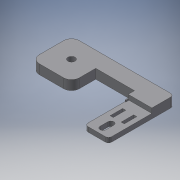
# Autodesk Inventor part: FiberMount
Saved by Autodesk Inventor 2019 (Build 230136000, 136)
## iProperties
Created: 2019-05-24
Part Number: FiberMount
Material: Generic
Document SubType Name: Modeling
Designer: aorfi
Density: 1 g/cm^3
Appearance: Default
Author: aorfi
Autodesk Inventor part; units mm, degrees
ref_plane "YZ Plane" through (0, 0, 0) normal (1, 0, 0) x (0, 1, 0)
ref_plane "XZ Plane" through (0, 0, 0) normal (0, 1, 0) x (-1, 0, 0)
ref_plane "XY Plane" through (0, 0, 0) normal (0, 0, 1) x (1, 0, 0)
sketch "Sketch1" plane through (0, 0, 0) normal (0, 1, 0) x (-1, 0, 0)
  line L0 (-7.5, 25) -> (7.5, 25)
  line L1 (7.5, 25) -> (7.5, -16.5)
  line L2 (7.5, -16.5) -> (-7.5, -16.5)
  line L3 (-7.5, -16.5) -> (-7.5, 25)
  line L4 (7.5, -16.5) -> (57.5, -16.5)
  line L5 (57.5, -16.5) -> (57.5, 8.9)
  line L6 (57.5, 8.9) -> (32.1, 8.9)
  line L7 (32.1, 8.9) -> (32.1, -6.5)
  line L8 (32.1, -6.5) -> (7.5, -6.5)
  point P0 (0, 0)
  point P1 (0, -16.5)
  point P2 (57.5, -3.8)
  dimension "d30" = 15
  dimension "d31" = 16.5
  dimension "d32" = 25
  dimension "d59" = 50
  dimension "d60" = 25.4
  dimension "d61" = 10
  dimension "d62" = 25.4
  constraints: 18 end point, 4 horizontal, 3 perpendicular, 2 midpoint, 2 parallel, 1 point on line, 1 vertical alignment
  measures "d30" distance of L0.start L0.end
  measures "d31" distance from line of L2 point (0, 0)
  measures "d32" distance from line of point (0, 0) L0
  measures "d59" distance between parallel lines of L5 L1
  measures "d60" distance between parallel lines of L4 L6
  measures "d61" distance between parallel lines of L4 L8
  measures "d62" distance between parallel lines of L5 L7
extrude "Extrusion1" add sketch "Sketch1" along normal mid plane 3
sketch "Sketch4" plane through (0, 1.5, 0) normal (0, 1, 0) x (1, 0, 0)
  line L0 (7.5, 2.5) -> (-7.5, 2.5)
  line L1 (7.5, 2.5) -> (7.5, 14.5)
  line L2 (-7.5, 6.5) -> (-7.5, 2.5)
  line L3 (7.5, -25) -> (7.5, 16.5) projected
  line L4 (-7.5, 6.5) -> (-7.5, -25) projected
  line L5 (-7.5, -25) -> (7.5, -25) projected
  line L6 (7.5, 16.5) -> (-57.5, 16.5) projected
  line L7 (7.5, 16.5) -> (-7.5, 16.5)
  line L8 (-7.5, -25) -> (7.5, -25) projected
  line L9 (7.5, -25) -> (7.5, 16.5) projected
  line L10 (7.5, 16.5) -> (-57.5, 16.5) projected
  line L11 (-57.5, 16.5) -> (-57.5, -8.9) projected
  line L12 (-57.5, -8.9) -> (-32.1, -8.9) projected
  line L13 (-32.1, -8.9) -> (-32.1, 6.5) projected
  line L14 (-32.1, 6.5) -> (-7.5, 6.5) projected
  line L15 (-7.5, 6.5) -> (-7.5, -25) projected
  point P0 (0, 0)
  dimension "d20" = 2.5
  constraints: 8 end point, 2 collinear, 2 horizontal, 2 other
  measures "d20" distance from line of L0 point (0, 0)
extrude "Extrusion3" add sketch "Sketch4" along normal blind 3 contours L0 L2 L14 L13 L12 L11 L6 L3 L1
sketch "Sketch5" plane through (0, 1.5, 0) normal (0, 1, 0) x (1, 0, 0)
  line L0 (-2.5, -14) -> (-4.5, -14)
  line L1 (-4.5, -14) -> (-4.5, -4)
  line L2 (-4.5, -4) -> (-2.5, -4)
  line L3 (-2.5, -4) -> (-2.5, -14)
  line L4 (-2.5, -14) -> (-4.5, -4) construction
  line L5 (-4.5, -14) -> (-2.5, -4) construction
  line L6 (4.5, -14) -> (2.5, -14)
  line L7 (2.5, -14) -> (2.5, -4)
  line L8 (2.5, -4) -> (4.5, -4)
  line L9 (4.5, -4) -> (4.5, -14)
  line L10 (4.5, -14) -> (2.5, -4) construction
  line L11 (2.5, -14) -> (4.5, -4) construction
  line L12 (-3.5, -9) -> (3.5, -9) construction
  point P0 (0, 0)
  point P1 (0, -9)
  dimension "d24" = 2
  dimension "d25" = 10
  dimension "d26" = 7
  dimension "d27" = 4
  constraints: 26 end point, 5 midpoint, 4 parallel, 3 horizontal, 2 equal length, 2 perpendicular, 1 point on line, 1 vertical alignment
  measures "d24" distance of L7.end L8.end
  measures "d25" distance of L8.end L6.start
  measures "d26" distance of L12.start L12.end
  measures "d27" distance from line of point (0, 0) L2
extrude "Extrusion4" cut sketch "Sketch5" against normal blind 2
sketch "Sketch6" plane through (0, 1.5, 0) normal (0, 1, 0) x (1, 0, 0)
  circle A0 centre (0, -16) radius 1.8986
  circle A1 centre (0, -21) radius 1.8986
  line L0 (1.8986, -21) -> (1.8986, -16)
  line L1 (-1.8986, -21) -> (-1.8986, -16)
  line L2 (-7.5, -25) -> (7.5, -25) projected
  point P0 (0, 0)
  dimension "d33" = 3.7973
  dimension "d36" = 3.7973
  dimension "d37" = 5
  dimension "d68" = 4
  constraints: 4 end point, 4 point on circle, 3 tangent, 2 centre point, 2 vertical alignment, 1 vertical
  measures "d33" diameter of A0
  measures "d36" diameter of A1
  measures "d37" distance of A0.centre A1.centre
  measures "d68" distance from line of A1.centre L2
extrude "Extrusion5" cut sketch "Sketch6" against normal through all
fillet "Fillet1" radius 5 3 edges at (-32.1, 1.5, 8.9) (-57.5, 1.5, 8.9) (-57.5, 1.5, -16.5)
fillet "Fillet2" radius 2 3 edges at (7.5, 1.5, -16.5) (7.5, 0, 25) (-7.5, 0, 25)
sketch "Sketch8" plane through (0, 1.5, 0) normal (0, 1, 0) x (1, 0, 0)
  line L0 (-7.5, 2.5) -> (7.5, 2.5) projected
  line L1 (-7.5, 2.5) -> (-7, 2.5)
  line L2 (-7, 2.5) -> (-7, 0.5)
  line L3 (-7, 0.5) -> (-7.5, 0.5)
  line L4 (-7.5, 0.5) -> (-7.5, 2.5)
  point P0 (0, 0)
  dimension "d74" = 0.5
  dimension "d75" = 2
  constraints: 8 end point, 2 parallel, 1 horizontal, 1 perpendicular
  measures "d74" distance of L2.end L3.end
  measures "d75" distance of L1.end L2.end
extrude "Extrusion6" add sketch "Sketch8" along normal blind 1
sketch "Sketch9" plane through (0, 4.5, 0) normal (0, 1, 0) x (1, 0, 0)
  line L0 (-57.5, 11.5) -> (-57.5, -3.9) projected
  line L1 (5.5, 16.5) -> (-52.5, 16.5) projected
  point P0 (0, 0)
  point P1 (-44.8, 3.8)
  dimension "d76" = 12.7
  dimension "d77" = 12.7
  measures "d76" distance from line of L0 point (-44.8, 3.8)
  measures "d77" distance from line of L1 point (-44.8, 3.8)
hole "Hole2" at (-44.8, 4.5, -3.8) direction (0, -1, 0) diameter 4.496 end through all clearance for "Flat Head Machine Screw (82)" size "#8" standard "Ansi Unified Screw Threads"
equation "\"d62\" = d60"
equation "\"d36\" = d33"
equation "\"d77\" = d76"
body "Solid1"
